Autodesk Fusion 360 part; units mm, degrees
(part 2 of 8)
  spline S13 degree 5 poles (-65.8949, -9.4893) (-65.8986, -9.4803) (-65.9059, -9.4622) (-65.917, -9.4352) (-65.9319, -9.3993) (-65.9507, -9.3546) (-65.9697, -9.3101) (-65.9889, -9.2657) (-66.0083, -9.2215) (-66.028, -9.1775) (-66.0478, -9.1337) (-66.0678, -9.09) (-66.088, -9.0466) (-66.1085, -9.0033) (-66.1291, -8.9602) (-66.1499, -8.9173) (-66.171, -8.8746) (-66.1922, -8.8321) (-66.2136, -8.7898) (-66.2353, -8.7476) (-66.2571, -8.7057) (-66.2792, -8.664) (-66.3015, -8.6224) (-66.3239, -8.5811) (-66.3466, -8.54) (-66.3695, -8.4991) (-66.3926, -8.4584) (-66.4159, -8.418) (-66.4394, -8.3777) (-66.4631, -8.3377) (-66.487, -8.2979) (-66.5111, -8.2583) (-66.5355, -8.2189) (-66.56, -8.1798) (-66.5848, -8.1409) (-66.6097, -8.1023) (-66.6349, -8.0638) (-66.6603, -8.0257) (-66.686, -7.9877) (-66.7118, -7.9501) (-66.7378, -7.9127) (-66.7641, -7.8755) (-66.7906, -7.8386) (-66.8173, -7.802) (-66.8443, -7.7657) (-66.8715, -7.7296) (-66.8989, -7.6938) (-66.9265, -7.6583) (-66.9543, -7.6231) (-66.9824, -7.5882) (-67.0107, -7.5535) (-67.0393, -7.5192) (-67.0681, -7.4853) (-67.0972, -7.4517) (-67.1265, -7.4185) (-67.1561, -7.3855) (-67.1859, -7.3529) (-67.216, -7.3206) (-67.2462, -7.2886) (-67.2768, -7.257) (-67.3076, -7.2258) (-67.3388, -7.1952) (-67.3704, -7.1651) (-67.4024, -7.1356) (-67.4347, -7.1066) (-67.4673, -7.078) (-67.5, -7.0497) (-67.5329, -7.0216) (-67.5661, -6.994) (-67.5997, -6.9671) (-67.6341, -6.9414) (-67.6624, -6.9221) (-67.6843, -6.9086) (-67.6991, -6.8999) (-67.7066, -6.8957) knots -1 -1 -1 -1 -1 -1 -0.98571429 -0.97142857 -0.95714286 -0.94285714 -0.92857143 -0.91428571 -0.9 -0.88571429 -0.87142857 -0.85714286 -0.84285714 -0.82857143 -0.81428571 -0.8 -0.78571429 -0.77142857 -0.75714286 -0.74285714 -0.72857143 -0.71428571 -0.7 -0.68571429 -0.67142857 -0.65714286 -0.64285714 -0.62857143 -0.61428571 -0.6 -0.58571429 -0.57142857 -0.55714286 -0.54285714 -0.52857143 -0.51428571 -0.5 -0.48571429 -0.47142857 -0.45714286 -0.44285714 -0.42857143 -0.41428571 -0.4 -0.38571429 -0.37142857 -0.35714286 -0.34285714 -0.32857143 -0.31428571 -0.3 -0.28571429 -0.27142857 -0.25714286 -0.24285714 -0.22857143 -0.21428571 -0.2 -0.18571429 -0.17142857 -0.15714286 -0.14285714 -0.12857143 -0.11428571 -0.1 -0.08571429 -0.07142857 -0.05714286 -0.04285714 -0.02857143 -0.01428571 0 0 0 0 0 0
  arc A44 (-68.6316, -5.3144) -> (-68.4437, -4.8923) centre (-80, 0) ccw
  spline S14 degree 5 poles (-66.6495, -4.5217) (-66.6414, -4.5244) (-66.6251, -4.5297) (-66.6004, -4.5368) (-66.5672, -4.545) (-66.525, -4.5533) (-66.4826, -4.5603) (-66.4398, -4.5664) (-66.397, -4.5721) (-66.354, -4.5775) (-66.3109, -4.5826) (-66.2678, -4.5872) (-66.2244, -4.5912) (-66.1809, -4.5946) (-66.1373, -4.5973) (-66.0935, -4.5993) (-66.0496, -4.6009) (-66.0055, -4.602) (-65.9614, -4.6027) (-65.9172, -4.603) (-65.873, -4.6029) (-65.8286, -4.6025) (-65.7842, -4.6016) (-65.7397, -4.6003) (-65.6951, -4.5986) (-65.6504, -4.5965) (-65.6057, -4.594) (-65.5609, -4.5911) (-65.516, -4.5879) (-65.4711, -4.5843) (-65.4261, -4.5803) (-65.381, -4.5761) (-65.336, -4.5714) (-65.2908, -4.5664) (-65.2456, -4.5611) (-65.2004, -4.5554) (-65.1551, -4.5494) (-65.1098, -4.5431) (-65.0644, -4.5364) (-65.019, -4.5294) (-64.9736, -4.5221) (-64.9281, -4.5145) (-64.8826, -4.5066) (-64.8371, -4.4983) (-64.7915, -4.4898) (-64.7459, -4.4809) (-64.7003, -4.4717) (-64.6547, -4.4623) (-64.609, -4.4525) (-64.5633, -4.4424) (-64.5176, -4.4321) (-64.4719, -4.4214) (-64.4262, -4.4105) (-64.3804, -4.3992) (-64.3346, -4.3877) (-64.2889, -4.3759) (-64.2431, -4.3638) (-64.1973, -4.3514) (-64.1515, -4.3387) (-64.1056, -4.3258) (-64.0598, -4.3125) (-64.014, -4.299) (-63.9682, -4.2853) (-63.9223, -4.2712) (-63.8765, -4.2569) (-63.8307, -4.2423) (-63.7848, -4.2274) (-63.739, -4.2123) (-63.6932, -4.1969) (-63.6474, -4.1812) (-63.6015, -4.1653) (-63.5649, -4.1523) (-63.5374, -4.1425) (-63.5191, -4.1359) (-63.5099, -4.1325) knots 0 0 0 0 0 0 0.01428571 0.02857143 0.04285714 0.05714286 0.07142857 0.08571429 0.1 0.11428571 0.12857143 0.14285714 0.15714286 0.17142857 0.18571429 0.2 0.21428571 0.22857143 0.24285714 0.25714286 0.27142857 0.28571429 0.3 0.31428571 0.32857143 0.34285714 0.35714286 0.37142857 0.38571429 0.4 0.41428571 0.42857143 0.44285714 0.45714286 0.47142857 0.48571429 0.5 0.51428571 0.52857143 0.54285714 0.55714286 0.57142857 0.58571429 0.6 0.61428571 0.62857143 0.64285714 0.65714286 0.67142857 0.68571429 0.7 0.71428571 0.72857143 0.74285714 0.75714286 0.77142857 0.78571429 0.8 0.81428571 0.82857143 0.84285714 0.85714286 0.87142857 0.88571429 0.9 0.91428571 0.92857143 0.94285714 0.95714286 0.97142857 0.98571429 1 1 1 1 1 1
  arc A45 (-63.5099, -4.1325) -> (-63.2547, -2.9318) centre (-80, 0) ccw
  spline S15 degree 5 poles (-63.2547, -2.9318) (-63.2617, -2.9251) (-63.2758, -2.9116) (-63.2969, -2.8914) (-63.3251, -2.8647) (-63.3605, -2.8315) (-63.3959, -2.7985) (-63.4315, -2.7658) (-63.4673, -2.7334) (-63.5031, -2.7011) (-63.539, -2.6692) (-63.5751, -2.6374) (-63.6112, -2.606) (-63.6475, -2.5747) (-63.6838, -2.5437) (-63.7203, -2.513) (-63.7569, -2.4826) (-63.7936, -2.4524) (-63.8304, -2.4224) (-63.8673, -2.3927) (-63.9043, -2.3633) (-63.9415, -2.3342) (-63.9787, -2.3053) (-64.016, -2.2767) (-64.0535, -2.2484) (-64.091, -2.2203) (-64.1286, -2.1925) (-64.1664, -2.165) (-64.2042, -2.1378) (-64.2422, -2.1109) (-64.2802, -2.0842) (-64.3184, -2.0579) (-64.3566, -2.0318) (-64.3949, -2.0061) (-64.4334, -1.9806) (-64.4719, -1.9555) (-64.5105, -1.9306) (-64.5493, -1.9061) (-64.5881, -1.8819) (-64.627, -1.858) (-64.666, -1.8344) (-64.7052, -1.8111) (-64.7444, -1.7882) (-64.7837, -1.7656) (-64.8231, -1.7434) (-64.8626, -1.7215) (-64.9021, -1.6999) (-64.9418, -1.6787) (-64.9816, -1.6579) (-65.0214, -1.6374) (-65.0614, -1.6173) (-65.1014, -1.5976) (-65.1416, -1.5783) (-65.1818, -1.5594) (-65.2221, -1.541) (-65.2626, -1.5229) (-65.3031, -1.5053) (-65.3436, -1.4879) (-65.3843, -1.471) (-65.4251, -1.4546) (-65.4659, -1.4387) (-65.5069, -1.4234) (-65.548, -1.4088) (-65.5892, -1.3948) (-65.6305, -1.3815) (-65.6719, -1.3686) (-65.7134, -1.356) (-65.7548, -1.3438) (-65.7964, -1.332) (-65.838, -1.3211) (-65.8799, -1.3116) (-65.9136, -1.3055) (-65.939, -1.302) (-65.9561, -1.3002) (-65.9646, -1.2994) knots -1 -1 -1 -1 -1 -1 -0.98571429 -0.97142857 -0.95714286 -0.94285714 -0.92857143 -0.91428571 -0.9 -0.88571429 -0.87142857 -0.85714286 -0.84285714 -0.82857143 -0.81428571 -0.8 -0.78571429 -0.77142857 -0.75714286 -0.74285714 -0.72857143 -0.71428571 -0.7 -0.68571429 -0.67142857 -0.65714286 -0.64285714 -0.62857143 -0.61428571 -0.6 -0.58571429 -0.57142857 -0.55714286 -0.54285714 -0.52857143 -0.51428571 -0.5 -0.48571429 -0.47142857 -0.45714286 -0.44285714 -0.42857143 -0.41428571 -0.4 -0.38571429 -0.37142857 -0.35714286 -0.34285714 -0.32857143 -0.31428571 -0.3 -0.28571429 -0.27142857 -0.25714286 -0.24285714 -0.22857143 -0.21428571 -0.2 -0.18571429 -0.17142857 -0.15714286 -0.14285714 -0.12857143 -0.11428571 -0.1 -0.08571429 -0.07142857 -0.05714286 -0.04285714 -0.02857143 -0.01428571 0 0 0 0 0 0
  arc A46 (-67.4529, -0.231) -> (-67.4529, 0.231) centre (-80, 0) ccw
  spline S16 degree 5 poles (-65.9646, 1.2994) (-65.9561, 1.3002) (-65.939, 1.302) (-65.9136, 1.3055) (-65.8799, 1.3116) (-65.838, 1.3211) (-65.7964, 1.332) (-65.7548, 1.3438) (-65.7134, 1.356) (-65.6719, 1.3686) (-65.6305, 1.3815) (-65.5892, 1.3948) (-65.548, 1.4088) (-65.5069, 1.4234) (-65.4659, 1.4387) (-65.4251, 1.4546) (-65.3843, 1.471) (-65.3436, 1.4879) (-65.3031, 1.5053) (-65.2626, 1.5229) (-65.2221, 1.541) (-65.1818, 1.5594) (-65.1416, 1.5783) (-65.1014, 1.5976) (-65.0614, 1.6173) (-65.0214, 1.6374) (-64.9816, 1.6579) (-64.9418, 1.6787) (-64.9021, 1.6999) (-64.8626, 1.7215) (-64.8231, 1.7434) (-64.7837, 1.7656) (-64.7444, 1.7882) (-64.7052, 1.8111) (-64.666, 1.8344) (-64.627, 1.858) (-64.5881, 1.8819) (-64.5493, 1.9061) (-64.5105, 1.9306) (-64.4719, 1.9555) (-64.4334, 1.9806) (-64.3949, 2.0061) (-64.3566, 2.0318) (-64.3184, 2.0579) (-64.2802, 2.0842) (-64.2422, 2.1109) (-64.2042, 2.1378) (-64.1664, 2.165) (-64.1286, 2.1925) (-64.091, 2.2203) (-64.0535, 2.2484) (-64.016, 2.2767) (-63.9787, 2.3053) (-63.9415, 2.3342) (-63.9043, 2.3633) (-63.8673, 2.3927) (-63.8304, 2.4224) (-63.7936, 2.4524) (-63.7569, 2.4826) (-63.7203, 2.513) (-63.6838, 2.5437) (-63.6475, 2.5747) (-63.6112, 2.606) (-63.5751, 2.6374) (-63.539, 2.6692) (-63.5031, 2.7011) (-63.4673, 2.7334) (-63.4315, 2.7658) (-63.3959, 2.7985) (-63.3605, 2.8315) (-63.3251, 2.8647) (-63.2969, 2.8914) (-63.2758, 2.9116) (-63.2617, 2.9251) (-63.2547, 2.9318) knots 0 0 0 0 0 0 0.01428571 0.02857143 0.04285714 0.05714286 0.07142857 0.08571429 0.1 0.11428571 0.12857143 0.14285714 0.15714286 0.17142857 0.18571429 0.2 0.21428571 0.22857143 0.24285714 0.25714286 0.27142857 0.28571429 0.3 0.31428571 0.32857143 0.34285714 0.35714286 0.37142857 0.38571429 0.4 0.41428571 0.42857143 0.44285714 0.45714286 0.47142857 0.48571429 0.5 0.51428571 0.52857143 0.54285714 0.55714286 0.57142857 0.58571429 0.6 0.61428571 0.62857143 0.64285714 0.65714286 0.67142857 0.68571429 0.7 0.71428571 0.72857143 0.74285714 0.75714286 0.77142857 0.78571429 0.8 0.81428571 0.82857143 0.84285714 0.85714286 0.87142857 0.88571429 0.9 0.91428571 0.92857143 0.94285714 0.95714286 0.97142857 0.98571429 1 1 1 1 1 1
  arc A47 (-63.2547, 2.9318) -> (-63.5099, 4.1325) centre (-80, 0) ccw
  spline S17 degree 5 poles (-63.5099, 4.1325) (-63.5191, 4.1359) (-63.5374, 4.1425) (-63.5649, 4.1523) (-63.6015, 4.1653) (-63.6474, 4.1812) (-63.6932, 4.1969) (-63.739, 4.2123) (-63.7848, 4.2274) (-63.8307, 4.2423) (-63.8765, 4.2569) (-63.9223, 4.2712) (-63.9682, 4.2853) (-64.014, 4.299) (-64.0598, 4.3125) (-64.1056, 4.3258) (-64.1515, 4.3387) (-64.1973, 4.3514) (-64.2431, 4.3638) (-64.2889, 4.3759) (-64.3346, 4.3877) (-64.3804, 4.3992) (-64.4262, 4.4105) (-64.4719, 4.4214) (-64.5176, 4.4321) (-64.5633, 4.4424) (-64.609, 4.4525) (-64.6547, 4.4623) (-64.7003, 4.4717) (-64.7459, 4.4809) (-64.7915, 4.4898) (-64.8371, 4.4983) (-64.8826, 4.5066) (-64.9281, 4.5145) (-64.9736, 4.5221) (-65.019, 4.5294) (-65.0644, 4.5364) (-65.1098, 4.5431) (-65.1551, 4.5494) (-65.2004, 4.5554) (-65.2456, 4.5611) (-65.2908, 4.5664) (-65.336, 4.5714) (-65.381, 4.5761) (-65.4261, 4.5803) (-65.4711, 4.5843) (-65.516, 4.5879) (-65.5609, 4.5911) (-65.6057, 4.594) (-65.6504, 4.5965) (-65.6951, 4.5986) (-65.7397, 4.6003) (-65.7842, 4.6016) (-65.8286, 4.6025) (-65.873, 4.6029) (-65.9172, 4.603) (-65.9614, 4.6027) (-66.0055, 4.602) (-66.0496, 4.6009) (-66.0935, 4.5993) (-66.1373, 4.5973) (-66.1809, 4.5946) (-66.2244, 4.5912) (-66.2678, 4.5872) (-66.3109, 4.5826) (-66.354, 4.5775) (-66.397, 4.5721) (-66.4398, 4.5664) (-66.4826, 4.5603) (-66.525, 4.5533) (-66.5672, 4.545) (-66.6004, 4.5368) (-66.6251, 4.5297) (-66.6414, 4.5244) (-66.6495, 4.5217) knots -1 -1 -1 -1 -1 -1 -0.98571429 -0.97142857 -0.95714286 -0.94285714 -0.92857143 -0.91428571 -0.9 -0.88571429 -0.87142857 -0.85714286 -0.84285714 -0.82857143 -0.81428571 -0.8 -0.78571429 -0.77142857 -0.75714286 -0.74285714 -0.72857143 -0.71428571 -0.7 -0.68571429 -0.67142857 -0.65714286 -0.64285714 -0.62857143 -0.61428571 -0.6 -0.58571429 -0.57142857 -0.55714286 -0.54285714 -0.52857143 -0.51428571 -0.5 -0.48571429 -0.47142857 -0.45714286 -0.44285714 -0.42857143 -0.41428571 -0.4 -0.38571429 -0.37142857 -0.35714286 -0.34285714 -0.32857143 -0.31428571 -0.3 -0.28571429 -0.27142857 -0.25714286 -0.24285714 -0.22857143 -0.21428571 -0.2 -0.18571429 -0.17142857 -0.15714286 -0.14285714 -0.12857143 -0.11428571 -0.1 -0.08571429 -0.07142857 -0.05714286 -0.04285714 -0.02857143 -0.01428571 0 0 0 0 0 0
  arc A48 (-68.4437, 4.8923) -> (-68.6316, 5.3144) centre (-80, 0) ccw
  spline S18 degree 5 poles (-67.7066, 6.8957) (-67.6991, 6.8999) (-67.6843, 6.9086) (-67.6624, 6.9221) (-67.6341, 6.9414) (-67.5997, 6.9671) (-67.5661, 6.994) (-67.5329, 7.0216) (-67.5, 7.0497) (-67.4673, 7.078) (-67.4347, 7.1066) (-67.4024, 7.1356) (-67.3704, 7.1651) (-67.3388, 7.1952) (-67.3076, 7.2258) (-67.2768, 7.257) (-67.2462, 7.2886) (-67.216, 7.3206) (-67.1859, 7.3529) (-67.1561, 7.3855) (-67.1265, 7.4185) (-67.0972, 7.4517) (-67.0681, 7.4853) (-67.0393, 7.5192) (-67.0107, 7.5535) (-66.9824, 7.5882) (-66.9543, 7.6231) (-66.9265, 7.6583) (-66.8989, 7.6938) (-66.8715, 7.7296) (-66.8443, 7.7657) (-66.8173, 7.802) (-66.7906, 7.8386) (-66.7641, 7.8755) (-66.7378, 7.9127) (-66.7118, 7.9501) (-66.686, 7.9877) (-66.6603, 8.0257) (-66.6349, 8.0638) (-66.6097, 8.1023) (-66.5848, 8.1409) (-66.56, 8.1798) (-66.5355, 8.2189) (-66.5111, 8.2583) (-66.487, 8.2979) (-66.4631, 8.3377) (-66.4394, 8.3777) (-66.4159, 8.418) (-66.3926, 8.4584) (-66.3695, 8.4991) (-66.3466, 8.54) (-66.3239, 8.5811) (-66.3015, 8.6224) (-66.2792, 8.664) (-66.2571, 8.7057) (-66.2353, 8.7476) (-66.2136, 8.7898) (-66.1922, 8.8321) (-66.171, 8.8746) (-66.1499, 8.9173) (-66.1291, 8.9602) (-66.1085, 9.0033) (-66.088, 9.0466) (-66.0678, 9.09) (-66.0478, 9.1337) (-66.028, 9.1775) (-66.0083, 9.2215) (-65.9889, 9.2657) (-65.9697, 9.3101) (-65.9507, 9.3546) (-65.9319, 9.3993) (-65.917, 9.4352) (-65.9059, 9.4622) (-65.8986, 9.4803) (-65.8949, 9.4893) knots 0 0 0 0 0 0 0.01428571 0.02857143 0.04285714 0.05714286 0.07142857 0.08571429 0.1 0.11428571 0.12857143 0.14285714 0.15714286 0.17142857 0.18571429 0.2 0.21428571 0.22857143 0.24285714 0.25714286 0.27142857 0.28571429 0.3 0.31428571 0.32857143 0.34285714 0.35714286 0.37142857 0.38571429 0.4 0.41428571 0.42857143 0.44285714 0.45714286 0.47142857 0.48571429 0.5 0.51428571 0.52857143 0.54285714 0.55714286 0.57142857 0.58571429 0.6 0.61428571 0.62857143 0.64285714 0.65714286 0.67142857 0.68571429 0.7 0.71428571 0.72857143 0.74285714 0.75714286 0.77142857 0.78571429 0.8 0.81428571 0.82857143 0.84285714 0.85714286 0.87142857 0.88571429 0.9 0.91428571 0.92857143 0.94285714 0.95714286 0.97142857 0.98571429 1 1 1 1 1 1
  arc A49 (-65.8949, 9.4893) -> (-66.6164, 10.4824) centre (-80, 0) ccw
  spline S19 degree 5 poles (-66.6164, 10.4824) (-66.6262, 10.4817) (-66.6456, 10.4803) (-66.6747, 10.4781) (-66.7134, 10.475) (-66.7618, 10.4709) (-66.81, 10.4666) (-66.8581, 10.4621) (-66.9061, 10.4572) (-66.9541, 10.4522) (-67.0019, 10.4469) (-67.0496, 10.4413) (-67.0972, 10.4355) (-67.1446, 10.4295) (-67.192, 10.4232) (-67.2392, 10.4166) (-67.2864, 10.4098) (-67.3334, 10.4027) (-67.3802, 10.3954) (-67.427, 10.3879) (-67.4736, 10.38) (-67.5201, 10.3719) (-67.5665, 10.3636) (-67.6127, 10.355) (-67.6588, 10.3461) (-67.7048, 10.337) (-67.7506, 10.3276) (-67.7963, 10.318) (-67.8419, 10.3081) (-67.8873, 10.2979) (-67.9325, 10.2875) (-67.9776, 10.2767) (-68.0226, 10.2658) (-68.0674, 10.2545) (-68.112, 10.243) (-68.1565, 10.2312) (-68.2008, 10.2191) (-68.245, 10.2067) (-68.2889, 10.1941) (-68.3327, 10.1811) (-68.3764, 10.1679) (-68.4198, 10.1544) (-68.4631, 10.1406) (-68.5062, 10.1265) (-68.5491, 10.1121) (-68.5918, 10.0974) (-68.6343, 10.0824) (-68.6766, 10.0671) (-68.7187, 10.0515) (-68.7606, 10.0356) (-68.8022, 10.0194) (-68.8437, 10.0028) (-68.8849, 9.9859) (-68.9258, 9.9686) (-68.9665, 9.951) (-69.007, 9.933) (-69.0472, 9.9147) (-69.0872, 9.8962) (-69.127, 9.8773) (-69.1665, 9.858) (-69.2057, 9.8383) (-69.2444, 9.8181) (-69.2828, 9.7973) (-69.3207, 9.776) (-69.3583, 9.7542) (-69.3956, 9.7321) (-69.4327, 9.7097) (-69.4695, 9.6871) (-69.506, 9.6641) (-69.542, 9.6404) (-69.5771, 9.6157) (-69.6042, 9.5947) (-69.6238, 9.5781) (-69.6366, 9.5667) (-69.6429, 9.5609) knots -1 -1 -1 -1 -1 -1 -0.98571429 -0.97142857 -0.95714286 -0.94285714 -0.92857143 -0.91428571 -0.9 -0.88571429 -0.87142857 -0.85714286 -0.84285714 -0.82857143 -0.81428571 -0.8 -0.78571429 -0.77142857 -0.75714286 -0.74285714 -0.72857143 -0.71428571 -0.7 -0.68571429 -0.67142857 -0.65714286 -0.64285714 -0.62857143 -0.61428571 -0.6 -0.58571429 -0.57142857 -0.55714286 -0.54285714 -0.52857143 -0.51428571 -0.5 -0.48571429 -0.47142857 -0.45714286 -0.44285714 -0.42857143 -0.41428571 -0.4 -0.38571429 -0.37142857 -0.35714286 -0.34285714 -0.32857143 -0.31428571 -0.3 -0.28571429 -0.27142857 -0.25714286 -0.24285714 -0.22857143 -0.21428571 -0.2 -0.18571429 -0.17142857 -0.15714286 -0.14285714 -0.12857143 -0.11428571 -0.1 -0.08571429 -0.07142857 -0.05714286 -0.04285714 -0.02857143 -0.01428571 0 0 0 0 0 0
  arc A50 (-71.4327, 9.1697) -> (-71.7761, 9.4789) centre (-80, 0) ccw
  spline S20 degree 5 poles (-71.5741, 11.2998) (-71.569, 11.3066) (-71.559, 11.3205) (-71.5445, 11.3418) (-71.5265, 11.3709) (-71.5055, 11.4084) (-71.4858, 11.4466) (-71.4667, 11.4854) (-71.4481, 11.5244) (-71.4297, 11.5636) (-71.4116, 11.603) (-71.3939, 11.6426) (-71.3766, 11.6826) (-71.36, 11.7229) (-71.3439, 11.7636) (-71.3284, 11.8046) (-71.3134, 11.8459) (-71.2987, 11.8874) (-71.2844, 11.9292) (-71.2705, 11.9711) (-71.2569, 12.0132) (-71.2436, 12.0555) (-71.2307, 12.098) (-71.2181, 12.1408) (-71.206, 12.1837) (-71.1942, 12.2269) (-71.1828, 12.2702) (-71.1717, 12.3137) (-71.1609, 12.3574) (-71.1504, 12.4012) (-71.1402, 12.4452) (-71.1304, 12.4894) (-71.1209, 12.5337) (-71.1117, 12.5782) (-71.1028, 12.6228) (-71.0942, 12.6676) (-71.0859, 12.7125) (-71.0779, 12.7575) (-71.0703, 12.8027) (-71.0629, 12.8481) (-71.0558, 12.8935) (-71.049, 12.9391) (-71.0425, 12.9849) (-71.0362, 13.0307) (-71.0303, 13.0767) (-71.0246, 13.1228) (-71.0193, 13.169) (-71.0142, 13.2154) (-71.0093, 13.2618) (-71.0048, 13.3084) (-71.0005, 13.355) (-70.9965, 13.4018) (-70.9928, 13.4487) (-70.9894, 13.4957) (-70.9862, 13.5428) (-70.9833, 13.59) (-70.9806, 13.6373) (-70.9783, 13.6846) (-70.9762, 13.7321) (-70.9743, 13.7797) (-70.9727, 13.8274) (-70.9714, 13.8751) (-70.9704, 13.923) (-70.9696, 13.9709) (-70.969, 14.0189) (-70.9687, 14.067) (-70.9687, 14.1152) (-70.969, 14.1635) (-70.9694, 14.2118) (-70.9702, 14.2602) (-70.9712, 14.3087) (-70.9722, 14.3476) (-70.9731, 14.3768) (-70.9737, 14.3962) (-70.974, 14.406) knots 0 0 0 0 0 0 0.01428571 0.02857143 0.04285714 0.05714286 0.07142857 0.08571429 0.1 0.11428571 0.12857143 0.14285714 0.15714286 0.17142857 0.18571429 0.2 0.21428571 0.22857143 0.24285714 0.25714286 0.27142857 0.28571429 0.3 0.31428571 0.32857143 0.34285714 0.35714286 0.37142857 0.38571429 0.4 0.41428571 0.42857143 0.44285714 0.45714286 0.47142857 0.48571429 0.5 0.51428571 0.52857143 0.54285714 0.55714286 0.57142857 0.58571429 0.6 0.61428571 0.62857143 0.64285714 0.65714286 0.67142857 0.68571429 0.7 0.71428571 0.72857143 0.74285714 0.75714286 0.77142857 0.78571429 0.8 0.81428571 0.82857143 0.84285714 0.85714286 0.87142857 0.88571429 0.9 0.91428571 0.92857143 0.94285714 0.95714286 0.97142857 0.98571429 1 1 1 1 1 1
  arc A51 (-70.974, 14.406) -> (-72.0371, 15.0197) centre (-80, 0) ccw
  spline S21 degree 5 poles (-72.0371, 15.0197) (-72.0457, 15.0151) (-72.0628, 15.0059) (-72.0885, 14.9921) (-72.1227, 14.9735) (-72.1652, 14.9502) (-72.2075, 14.9266) (-72.2496, 14.9028) (-72.2915, 14.8789) (-72.3332, 14.8548) (-72.3748, 14.8305) (-72.4161, 14.806) (-72.4572, 14.7814) (-72.4981, 14.7565) (-72.5388, 14.7315) (-72.5793, 14.7063) (-72.6196, 14.6809) (-72.6596, 14.6554) (-72.6995, 14.6296) (-72.7391, 14.6037) (-72.7785, 14.5776) (-72.8177, 14.5513) (-72.8567, 14.5248) (-72.8954, 14.4981) (-72.9339, 14.4713) (-72.9722, 14.4443) (-73.0103, 14.417) (-73.0481, 14.3896) (-73.0857, 14.3621) (-73.123, 14.3343) (-73.1601, 14.3063) (-73.1969, 14.2782) (-73.2335, 14.2499) (-73.2699, 14.2214) (-73.306, 14.1927) (-73.3418, 14.1638) (-73.3774, 14.1348) (-73.4127, 14.1055) (-73.4477, 14.0761) (-73.4825, 14.0464) (-73.517, 14.0166) (-73.5512, 13.9866) (-73.5851, 13.9564) (-73.6187, 13.926) (-73.652, 13.8954) (-73.685, 13.8646) (-73.7178, 13.8336) (-73.7502, 13.8024) (-73.7823, 13.7711) (-73.8141, 13.7395) (-73.8456, 13.7077) (-73.8767, 13.6757) (-73.9075, 13.6435) (-73.9378, 13.611) (-73.9678, 13.5784) (-73.9975, 13.5455) (-74.0268, 13.5125) (-74.0558, 13.4792) (-74.0845, 13.4458) (-74.1127, 13.4121) (-74.1405, 13.3782) (-74.1677, 13.3439) (-74.1943, 13.3094) (-74.2203, 13.2745) (-74.2457, 13.2393) (-74.2708, 13.2039) (-74.2956, 13.1684) (-74.32, 13.1327) (-74.344, 13.0969) (-74.3673, 13.0606) (-74.3893, 13.0237) (-74.4054, 12.9935) (-74.4166, 12.9704) (-74.4237, 12.9548) (-74.4271, 12.9469) knots -1 -1 -1 -1 -1 -1 -0.98571429 -0.97142857 -0.95714286 -0.94285714 -0.92857143 -0.91428571 -0.9 -0.88571429 -0.87142857 -0.85714286 -0.84285714 -0.82857143 -0.81428571 -0.8 -0.78571429 -0.77142857 -0.75714286 -0.74285714 -0.72857143 -0.71428571 -0.7 -0.68571429 -0.67142857 -0.65714286 -0.64285714 -0.62857143 -0.61428571 -0.6 -0.58571429 -0.57142857 -0.55714286 -0.54285714 -0.52857143 -0.51428571 -0.5 -0.48571429 -0.47142857 -0.45714286 -0.44285714 -0.42857143 -0.41428571 -0.4 -0.38571429 -0.37142857 -0.35714286 -0.34285714 -0.32857143 -0.31428571 -0.3 -0.28571429 -0.27142857 -0.25714286 -0.24285714 -0.22857143 -0.21428571 -0.2 -0.18571429 -0.17142857 -0.15714286 -0.14285714 -0.12857143 -0.11428571 -0.1 -0.08571429 -0.07142857 -0.05714286 -0.04285714 -0.02857143 -0.01428571 0 0 0 0 0 0
  arc A52 (-75.903, 11.8616) -> (-76.3425, 12.0044) centre (-80, 0) ccw
  spline S22 degree 5 poles (-76.8986, 13.75) (-76.8967, 13.7583) (-76.8932, 13.7751) (-76.8887, 13.8004) (-76.884, 13.8343) (-76.8801, 13.8771) (-76.8776, 13.9201) (-76.876, 13.9632) (-76.8748, 14.0064) (-76.874, 14.0497) (-76.8734, 14.0931) (-76.8734, 14.1365) (-76.8739, 14.18) (-76.8751, 14.2236) (-76.877, 14.2673) (-76.8795, 14.3111) (-76.8825, 14.3549) (-76.8861, 14.3988) (-76.89, 14.4428) (-76.8943, 14.4867) (-76.8989, 14.5308) (-76.904, 14.5748) (-76.9095, 14.6189) (-76.9155, 14.6631) (-76.9218, 14.7072) (-76.9286, 14.7514) (-76.9358, 14.7957) (-76.9433, 14.8399) (-76.9512, 14.8842) (-76.9595, 14.9285) (-76.9681, 14.9729) (-76.9771, 15.0172) (-76.9864, 15.0616) (-76.9961, 15.1059) (-77.0061, 15.1503) (-77.0165, 15.1947) (-77.0272, 15.2391) (-77.0383, 15.2835) (-77.0496, 15.3279) (-77.0613, 15.3724) (-77.0733, 15.4168) (-77.0857, 15.4612) (-77.0983, 15.5056) (-77.1113, 15.5501) (-77.1245, 15.5945) (-77.1381, 15.6389) (-77.152, 15.6833) (-77.1662, 15.7277) (-77.1807, 15.7721) (-77.1955, 15.8165) (-77.2106, 15.8608) (-77.2259, 15.9052) (-77.2416, 15.9495) (-77.2576, 15.9939) (-77.2738, 16.0382) (-77.2904, 16.0825) (-77.3072, 16.1268) (-77.3243, 16.171) (-77.3417, 16.2152) (-77.3593, 16.2595) (-77.3773, 16.3036) (-77.3955, 16.3478) (-77.414, 16.3919) (-77.4328, 16.4361) (-77.4518, 16.4801) (-77.4711, 16.5242) (-77.4907, 16.5682) (-77.5105, 16.6122) (-77.5306, 16.6562) (-77.551, 16.7001) (-77.5716, 16.744) (-77.5884, 16.7791) (-77.601, 16.8054) (-77.6095, 16.8229) (-77.6138, 16.8317) knots 0 0 0 0 0 0 0.01428571 0.02857143 0.04285714 0.05714286 0.07142857 0.08571429 0.1 0.11428571 0.12857143 0.14285714 0.15714286 0.17142857 0.18571429 0.2 0.21428571 0.22857143 0.24285714 0.25714286 0.27142857 0.28571429 0.3 0.31428571 0.32857143 0.34285714 0.35714286 0.37142857 0.38571429 0.4 0.41428571 0.42857143 0.44285714 0.45714286 0.47142857 0.48571429 0.5 0.51428571 0.52857143 0.54285714 0.55714286 0.57142857 0.58571429 0.6 0.61428571 0.62857143 0.64285714 0.65714286 0.67142857 0.68571429 0.7 0.71428571 0.72857143 0.74285714 0.75714286 0.77142857 0.78571429 0.8 0.81428571 0.82857143 0.84285714 0.85714286 0.87142857 0.88571429 0.9 0.91428571 0.92857143 0.94285714 0.95714286 0.97142857 0.98571429 1 1 1 1 1 1
  arc A53 (-77.6138, 16.8317) -> (-78.8346, 16.96) centre (-80, 0) ccw
  spline S23 degree 5 poles (-78.8346, 16.96) (-78.8406, 16.9523) (-78.8525, 16.9369) (-78.8704, 16.9138) (-78.894, 16.883) (-78.9233, 16.8444) (-78.9524, 16.8056) (-78.9812, 16.7668) (-79.0098, 16.7279) (-79.0381, 16.6889) (-79.0661, 16.6498) (-79.0939, 16.6107) (-79.1214, 16.5714) (-79.1487, 16.5321) (-79.1757, 16.4927) (-79.2024, 16.4532) (-79.2289, 16.4136) (-79.2551, 16.3739) (-79.281, 16.3342) (-79.3067, 16.2944) (-79.3321, 16.2545) (-79.3572, 16.2145) (-79.382, 16.1745) (-79.4066, 16.1344) (-79.4308, 16.0942) (-79.4548, 16.0539) (-79.4785, 16.0136) (-79.5019, 15.9732) (-79.525, 15.9327) (-79.5478, 15.8922) (-79.5704, 15.8515) (-79.5926, 15.8109) (-79.6145, 15.7701) (-79.6361, 15.7293) (-79.6574, 15.6884) (-79.6784, 15.6474) (-79.699, 15.6064) (-79.7194, 15.5653) (-79.7394, 15.5242) (-79.7591, 15.483) (-79.7785, 15.4417) (-79.7975, 15.4004) (-79.8162, 15.359) (-79.8346, 15.3175) (-79.8526, 15.276) (-79.8702, 15.2345) (-79.8875, 15.1928) (-79.9045, 15.1512) (-79.9211, 15.1094) (-79.9373, 15.0677) (-79.9531, 15.0258) (-79.9685, 14.9839) (-79.9835, 14.942) (-79.998, 14.9) (-80.0122, 14.858) (-80.0259, 14.8159) (-80.0392, 14.7738) (-80.0522, 14.7316) (-80.0648, 14.6894) (-80.0769, 14.6471) (-80.0884, 14.6049) (-80.0994, 14.5625) (-80.1096, 14.5201) (-80.1192, 14.4777) (-80.1281, 14.4352) (-80.1366, 14.3927) (-80.1448, 14.3501) (-80.1526, 14.3076) (-80.16, 14.2651) (-80.1665, 14.2225) (-80.1716, 14.1799) (-80.1741, 14.1457) (-80.1749, 14.12) (-80.1749, 14.1029) (-80.1748, 14.0943) knots -1 -1 -1 -1 -1 -1 -0.98571429 -0.97142857 -0.95714286 -0.94285714 -0.92857143 -0.91428571 -0.9 -0.88571429 -0.87142857 -0.85714286 -0.84285714 -0.82857143 -0.81428571 -0.8 -0.78571429 -0.77142857 -0.75714286 -0.74285714 -0.72857143 -0.71428571 -0.7 -0.68571429 -0.67142857 -0.65714286 -0.64285714 -0.62857143 -0.61428571 -0.6 -0.58571429 -0.57142857 -0.55714286 -0.54285714 -0.52857143 -0.51428571 -0.5 -0.48571429 -0.47142857 -0.45714286 -0.44285714 -0.42857143 -0.41428571 -0.4 -0.38571429 -0.37142857 -0.35714286 -0.34285714 -0.32857143 -0.31428571 -0.3 -0.28571429 -0.27142857 -0.25714286 -0.24285714 -0.22857143 -0.21428571 -0.2 -0.18571429 -0.17142857 -0.15714286 -0.14285714 -0.12857143 -0.11428571 -0.1 -0.08571429 -0.07142857 -0.05714286 -0.04285714 -0.02857143 -0.01428571 0 0 0 0 0 0
  arc A54 (-81.0818, 12.5025) -> (-81.5413, 12.4542) centre (-80, 0) ccw
  spline S24 degree 5 poles (-82.7594, 13.8227) (-82.761, 13.8311) (-82.7646, 13.8478) (-82.7708, 13.8728) (-82.7804, 13.9057) (-82.7942, 13.9463) (-82.8094, 13.9866) (-82.8254, 14.0267) (-82.8419, 14.0666) (-82.8588, 14.1065) (-82.8759, 14.1464) (-82.8935, 14.1861) (-82.9117, 14.2256) (-82.9305, 14.2649) (-82.95, 14.3041) (-82.9701, 14.3431) (-82.9907, 14.3819) (-83.0118, 14.4205) (-83.0333, 14.4591) (-83.0551, 14.4975) (-83.0772, 14.5358) (-83.0998, 14.574) (-83.1228, 14.6121) (-83.1461, 14.65) (-83.1699, 14.6877) (-83.1941, 14.7254) (-83.2186, 14.7629) (-83.2435, 14.8002) (-83.2688, 14.8375) (-83.2944, 14.8746) (-83.3203, 14.9116) (-83.3465, 14.9484) (-83.3731, 14.9851) (-83.3999, 15.0217) (-83.4272, 15.0582) (-83.4547, 15.0945) (-83.4825, 15.1308) (-83.5107, 15.1668) (-83.5391, 15.2028) (-83.5679, 15.2386) (-83.5969, 15.2743) (-83.6263, 15.3099) (-83.6559, 15.3453) (-83.6858, 15.3806) (-83.716, 15.4158) (-83.7464, 15.4509) (-83.7772, 15.4858) (-83.8082, 15.5206) (-83.8395, 15.5552) (-83.8711, 15.5898) (-83.9029, 15.6242) (-83.935, 15.6584) (-83.9673, 15.6926) (-84, 15.7266) (-84.0328, 15.7604) (-84.066, 15.7942) (-84.0993, 15.8278) (-84.133, 15.8613) (-84.1668, 15.8946) (-84.201, 15.9278) (-84.2353, 15.9609) (-84.2699, 15.9938) (-84.3048, 16.0266) (-84.3399, 16.0593) (-84.3752, 16.0918) (-84.4107, 16.1242) (-84.4465, 16.1565) (-84.4826, 16.1886) (-84.5188, 16.2206) (-84.5553, 16.2524) (-84.592, 16.2841) (-84.6215, 16.3094) (-84.6438, 16.3283) (-84.6587, 16.3408) (-84.6661, 16.3471) knots 0 0 0 0 0 0 0.01428571 0.02857143 0.04285714 0.05714286 0.07142857 0.08571429 0.1 0.11428571 0.12857143 0.14285714 0.15714286 0.17142857 0.18571429 0.2 0.21428571 0.22857143 0.24285714 0.25714286 0.27142857 0.28571429 0.3 0.31428571 0.32857143 0.34285714 0.35714286 0.37142857 0.38571429 0.4 0.41428571 0.42857143 0.44285714 0.45714286 0.47142857 0.48571429 0.5 0.51428571 0.52857143 0.54285714 0.55714286 0.57142857 0.58571429 0.6 0.61428571 0.62857143 0.64285714 0.65714286 0.67142857 0.68571429 0.7 0.71428571 0.72857143 0.74285714 0.75714286 0.77142857 0.78571429 0.8 0.81428571 0.82857143 0.84285714 0.85714286 0.87142857 0.88571429 0.9 0.91428571 0.92857143 0.94285714 0.95714286 0.97142857 0.98571429 1 1 1 1 1 1
  arc A55 (-84.6661, 16.3471) -> (-85.8336, 15.9678) centre (-80, 0) ccw
  spline S25 degree 5 poles (-85.8336, 15.9678) (-85.8359, 15.9583) (-85.8406, 15.9394) (-85.8475, 15.911) (-85.8566, 15.8732) (-85.8676, 15.826) (-85.8784, 15.7788) (-85.8889, 15.7316) (-85.8992, 15.6845) (-85.9092, 15.6373) (-85.9189, 15.5902) (-85.9284, 15.5431) (-85.9376, 15.4961) (-85.9465, 15.4491) (-85.9551, 15.4021) (-85.9635, 15.3551) (-85.9716, 15.3082) (-85.9794, 15.2613) (-85.9869, 15.2145) (-85.9942, 15.1677) (-86.0011, 15.1209) (-86.0078, 15.0742) (-86.0142, 15.0275) (-86.0203, 14.9809) (-86.0261, 14.9343) (-86.0317, 14.8877) (-86.0369, 14.8413) (-86.0419, 14.7948) (-86.0465, 14.7484) (-86.0509, 14.7021) (-86.0549, 14.6559) (-86.0586, 14.6096) (-86.0621, 14.5635) (-86.0652, 14.5174) (-86.068, 14.4714) (-86.0706, 14.4255) (-86.0728, 14.3796) (-86.0746, 14.3338) (-86.0762, 14.288) (-86.0775, 14.2424) (-86.0784, 14.1968) (-86.0789, 14.1513) (-86.0792, 14.1059) (-86.0791, 14.0605) (-86.0786, 14.0153) (-86.0779, 13.9702) (-86.0767, 13.9251) (-86.0753, 13.8801) (-86.0734, 13.8353) (-86.0713, 13.7905) (-86.0687, 13.7459) (-86.0657, 13.7013) (-86.0624, 13.6569) (-86.0586, 13.6126) (-86.0544, 13.5685) (-86.0498, 13.5245) (-86.0449, 13.4805) (-86.0396, 13.4368) (-86.0339, 13.3931) (-86.0278, 13.3496) (-86.0211, 13.3062) (-86.0139, 13.2631) (-86.006, 13.2202) (-85.9974, 13.1775) (-85.9883, 13.1351) (-85.9788, 13.0928) (-85.969, 13.0506) (-85.9589, 13.0086) (-85.9483, 12.9667) (-85.9369, 12.9252) (-85.9242, 12.8842) (-85.9126, 12.8519) (-85.9029, 12.8282) (-85.896, 12.8125) (-85.8924, 12.8047) knots -1 -1 -1 -1 -1 -1 -0.98571429 -0.97142857 -0.95714286 -0.94285714 -0.92857143 -0.91428571 -0.9 -0.88571429 -0.87142857 -0.85714286 -0.84285714 -0.82857143 -0.81428571 -0.8 -0.78571429 -0.77142857 -0.75714286 -0.74285714 -0.72857143 -0.71428571 -0.7 -0.68571429 -0.67142857 -0.65714286 -0.64285714 -0.62857143 -0.61428571 -0.6 -0.58571429 -0.57142857 -0.55714286 -0.54285714 -0.52857143 -0.51428571 -0.5 -0.48571429 -0.47142857 -0.45714286 -0.44285714 -0.42857143 -0.41428571 -0.4 -0.38571429 -0.37142857 -0.35714286 -0.34285714 -0.32857143 -0.31428571 -0.3 -0.28571429 -0.27142857 -0.25714286 -0.24285714 -0.22857143 -0.21428571 -0.2 -0.18571429 -0.17142857 -0.15714286 -0.14285714 -0.12857143 -0.11428571 -0.1 -0.08571429 -0.07142857 -0.05714286 -0.04285714 -0.02857143 -0.01428571 0 0 0 0 0 0
  arc A56 (-86.0735, 10.9816) -> (-86.4736, 10.7506) centre (-80, 0) ccw
  spline S26 degree 5 poles (-88.143, 11.5053) (-88.1479, 11.5123) (-88.1581, 11.5261) (-88.1738, 11.5464) (-88.1959, 11.5726) (-88.2251, 11.6041) (-88.2554, 11.6347) (-88.2863, 11.6648) (-88.3177, 11.6946) (-88.3493, 11.7242) (-88.3811, 11.7536) (-88.4134, 11.7827) (-88.446, 11.8114) (-88.4792, 11.8397) (-88.513, 11.8676) (-88.5472, 11.895) (-88.5818, 11.922) (-88.6168, 11.9488) (-88.6521, 11.9753) (-88.6876, 12.0015) (-88.7235, 12.0275) (-88.7596, 12.0532) (-88.796, 12.0786) (-88.8328, 12.1038) (-88.8699, 12.1286) (-88.9073, 12.1531) (-88.945, 12.1774) (-88.9829, 12.2014) (-89.0211, 12.2252) (-89.0596, 12.2487) (-89.0983, 12.2719) (-89.1372, 12.2949) (-89.1764, 12.3177) (-89.2159, 12.3402) (-89.2556, 12.3624) (-89.2955, 12.3844) (-89.3357, 12.4062) (-89.3761, 12.4277) (-89.4167, 12.4489) (-89.4575, 12.47) (-89.4986, 12.4908) (-89.5398, 12.5113) (-89.5813, 12.5317) (-89.623, 12.5518) (-89.6649, 12.5716) (-89.707, 12.5913) (-89.7493, 12.6106) (-89.7918, 12.6298) (-89.8345, 12.6487) (-89.8773, 12.6675) (-89.9204, 12.6859) (-89.9637, 12.7042) (-90.0071, 12.7222) (-90.0507, 12.74) (-90.0945, 12.7576) (-90.1385, 12.7749) (-90.1827, 12.7921) (-90.227, 12.809) (-90.2715, 12.8256) (-90.3162, 12.8421) (-90.361, 12.8583) (-90.406, 12.8743) (-90.4512, 12.8901) (-90.4966, 12.9057) (-90.5421, 12.9211) (-90.5877, 12.9362) (-90.6335, 12.9511) (-90.6795, 12.9658) (-90.7256, 12.9803) (-90.7719, 12.9945) (-90.8183, 13.0085) (-90.8556, 13.0196) (-90.8836, 13.0278) (-90.9023, 13.0332) (-90.9117, 13.0359) knots 0 0 0 0 0 0 0.01428571 0.02857143 0.04285714 0.05714286 0.07142857 0.08571429 0.1 0.11428571 0.12857143 0.14285714 0.15714286 0.17142857 0.18571429 0.2 0.21428571 0.22857143 0.24285714 0.25714286 0.27142857 0.28571429 0.3 0.31428571 0.32857143 0.34285714 0.35714286 0.37142857 0.38571429 0.4 0.41428571 0.42857143 0.44285714 0.45714286 0.47142857 0.48571429 0.5 0.51428571 0.52857143 0.54285714 0.55714286 0.57142857 0.58571429 0.6 0.61428571 0.62857143 0.64285714 0.65714286 0.67142857 0.68571429 0.7 0.71428571 0.72857143 0.74285714 0.75714286 0.77142857 0.78571429 0.8 0.81428571 0.82857143 0.84285714 0.85714286 0.87142857 0.88571429 0.9 0.91428571 0.92857143 0.94285714 0.95714286 0.97142857 0.98571429 1 1 1 1 1 1
  arc A57 (-90.9117, 13.0359) -> (-91.8239, 12.2145) centre (-80, 0) ccw
  spline S27 degree 5 poles (-91.8239, 12.2145) (-91.8222, 12.2049) (-91.8188, 12.1858) (-91.8136, 12.1571) (-91.8065, 12.1188) (-91.7974, 12.0712) (-91.788, 12.0237) (-91.7784, 11.9763) (-91.7686, 11.929) (-91.7586, 11.8819) (-91.7483, 11.8349) (-91.7378, 11.7881) (-91.7271, 11.7413) (-91.7161, 11.6948) (-91.7049, 11.6483) (-91.6934, 11.602) (-91.6817, 11.5559) (-91.6698, 11.5099) (-91.6576, 11.464) (-91.6452, 11.4183) (-91.6325, 11.3728) (-91.6196, 11.3274) (-91.6065, 11.2821) (-91.5931, 11.237) (-91.5795, 11.1921) (-91.5656, 11.1473) (-91.5515, 11.1027) (-91.5371, 11.0583) (-91.5225, 11.014) (-91.5076, 10.97) (-91.4925, 10.926) (-91.4771, 10.8823) (-91.4615, 10.8387) (-91.4456, 10.7954) (-91.4295, 10.7522) (-91.4131, 10.7092) (-91.3964, 10.6664) (-91.3795, 10.6238) (-91.3624, 10.5813) (-91.3449, 10.5391) (-91.3272, 10.4971) (-91.3092, 10.4553) (-91.291, 10.4137) (-91.2725, 10.3724) (-91.2537, 10.3312) (-91.2346, 10.2903) (-91.2152, 10.2496) (-91.1956, 10.2091) (-91.1757, 10.1689) (-91.1555, 10.1289) (-91.135, 10.0891) (-91.1142, 10.0496) (-91.093, 10.0104) (-91.0716, 9.9715) (-91.0498, 9.9329) (-91.0277, 9.8945) (-91.0053, 9.8564) (-90.9827, 9.8186) (-90.9597, 9.781) (-90.9364, 9.7437) (-90.9127, 9.7068) (-90.8885, 9.6704) (-90.8639, 9.6344) (-90.8387, 9.5989) (-90.8131, 9.5638) (-90.7872, 9.529) (-90.7611, 9.4945) (-90.7347, 9.4602) (-90.7081, 9.4263) (-90.6808, 9.393) (-90.6525, 9.3607) (-90.6288, 9.336) (-90.6102, 9.3182) (-90.5975, 9.3067) (-90.5911, 9.301) knots -1 -1 -1 -1 -1 -1 -0.98571429 -0.97142857 -0.95714286 -0.94285714 -0.92857143 -0.91428571 -0.9 -0.88571429 -0.87142857 -0.85714286 -0.84285714 -0.82857143 -0.81428571 -0.8 -0.78571429 -0.77142857 -0.75714286 -0.74285714 -0.72857143 -0.71428571 -0.7 -0.68571429 -0.67142857 -0.65714286 -0.64285714 -0.62857143 -0.61428571 -0.6 -0.58571429 -0.57142857 -0.55714286 -0.54285714 -0.52857143 -0.51428571 -0.5 -0.48571429 -0.47142857 -0.45714286 -0.44285714 -0.42857143 -0.41428571 -0.4 -0.38571429 -0.37142857 -0.35714286 -0.34285714 -0.32857143 -0.31428571 -0.3 -0.28571429 -0.27142857 -0.25714286 -0.24285714 -0.22857143 -0.21428571 -0.2 -0.18571429 -0.17142857 -0.15714286 -0.14285714 -0.12857143 -0.11428571 -0.1 -0.08571429 -0.07142857 -0.05714286 -0.04285714 -0.02857143 -0.01428571 0 0 0 0 0 0
  arc A58 (-90.015, 7.5619) -> (-90.2866, 7.1881) centre (-80, 0) ccw
  spline S28 degree 5 poles (-92.1186, 7.1986) (-92.126, 7.2029) (-92.1409, 7.2115) (-92.1635, 7.2236) (-92.1943, 7.2385) (-92.2338, 7.2554) (-92.2739, 7.2711) (-92.3144, 7.286) (-92.3552, 7.3005) (-92.3961, 7.3146) (-92.4372, 7.3285) (-92.4784, 7.342) (-92.52, 7.355) (-92.5618, 7.3673) (-92.604, 7.379) (-92.6464, 7.3902) (-92.689, 7.4008) (-92.7318, 7.411) (-92.7748, 7.4209) (-92.818, 7.4304) (-92.8613, 7.4395) (-92.9048, 7.4483) (-92.9484, 7.4567) (-92.9922, 7.4647) (-93.0362, 7.4723) (-93.0803, 7.4795) (-93.1246, 7.4864) (-93.1691, 7.4929) (-93.2136, 7.499) (-93.2583, 7.5048) (-93.3031, 7.5103) (-93.3481, 7.5155) (-93.3931, 7.5204) (-93.4383, 7.5249) (-93.4836, 7.529) (-93.5291, 7.5329) (-93.5746, 7.5364) (-93.6203, 7.5397) (-93.666, 7.5426) (-93.7119, 7.5452) (-93.7578, 7.5475) (-93.8039, 7.5495) (-93.8501, 7.5512) (-93.8963, 7.5526) (-93.9427, 7.5537) (-93.9891, 7.5545) (-94.0356, 7.555) (-94.0822, 7.5552) (-94.1289, 7.5552) (-94.1757, 7.5548) (-94.2226, 7.5542) (-94.2695, 7.5533) (-94.3165, 7.5521) (-94.3636, 7.5506) (-94.4108, 7.5488) (-94.458, 7.5468) (-94.5053, 7.5445) (-94.5527, 7.5419) (-94.6001, 7.539) (-94.6477, 7.5359) (-94.6952, 7.5325) (-94.7429, 7.5288) (-94.7906, 7.5248) (-94.8383, 7.5206) (-94.8861, 7.5161) (-94.934, 7.5114) (-94.9819, 7.5064) (-95.0299, 7.5011) (-95.0779, 7.4955) (-95.126, 7.4897) (-95.1741, 7.4837) (-95.2126, 7.4786) (-95.2416, 7.4747) (-95.2609, 7.4721) (-95.2705, 7.4707) knots 0 0 0 0 0 0 0.01428571 0.02857143 0.04285714 0.05714286 0.07142857 0.08571429 0.1 0.11428571 0.12857143 0.14285714 0.15714286 0.17142857 0.18571429 0.2 0.21428571 0.22857143 0.24285714 0.25714286 0.27142857 0.28571429 0.3 0.31428571 0.32857143 0.34285714 0.35714286 0.37142857 0.38571429 0.4 0.41428571 0.42857143 0.44285714 0.45714286 0.47142857 0.48571429 0.5 0.51428571 0.52857143 0.54285714 0.55714286 0.57142857 0.58571429 0.6 0.61428571 0.62857143 0.64285714 0.65714286 0.67142857 0.68571429 0.7 0.71428571 0.72857143 0.74285714 0.75714286 0.77142857 0.78571429 0.8 0.81428571 0.82857143 0.84285714 0.85714286 0.87142857 0.88571429 0.9 0.91428571 0.92857143 0.94285714 0.95714286 0.97142857 0.98571429 1 1 1 1 1 1
  arc A59 (-95.2705, 7.4707) -> (-95.7698, 6.3493) centre (-80, 0) ccw
  spline S29 degree 5 poles (-95.7698, 6.3493) (-95.7643, 6.3412) (-95.7534, 6.3251) (-95.7369, 6.301) (-95.7149, 6.269) (-95.6872, 6.2292) (-95.6594, 6.1896) (-95.6313, 6.1502) (-95.6032, 6.111) (-95.5748, 6.072) (-95.5463, 6.0333) (-95.5177, 5.9947) (-95.4888, 5.9564) (-95.4599, 5.9183) (-95.4307, 5.8805) (-95.4014, 5.8428) (-95.372, 5.8054) (-95.3424, 5.7683) (-95.3126, 5.7313) (-95.2827, 5.6946) (-95.2526, 5.6582) (-95.2223, 5.6219) (-95.1919, 5.5859) (-95.1613, 5.5502) (-95.1306, 5.5147) (-95.0997, 5.4794) (-95.0687, 5.4444) (-95.0375, 5.4097) (-95.0061, 5.3752) (-94.9746, 5.341) (-94.9429, 5.307) (-94.9111, 5.2733) (-94.8791, 5.2399) (-94.847, 5.2067) (-94.8147, 5.1738) (-94.7822, 5.1412) (-94.7496, 5.1089) (-94.7168, 5.0768) (-94.6838, 5.0451) (-94.6507, 5.0136) (-94.6175, 4.9824) (-94.5841, 4.9515) (-94.5505, 4.9209) (-94.5167, 4.8907) (-94.4828, 4.8608) (-94.4487, 4.8311) (-94.4145, 4.8018) (-94.3801, 4.7728) (-94.3455, 4.7442) (-94.3108, 4.7158) (-94.2759, 4.6878) (-94.2408, 4.6602) (-94.2056, 4.633) (-94.1702, 4.6062) (-94.1345, 4.5798) (-94.0988, 4.5537) (-94.0628, 4.528) (-94.0267, 4.5027) (-93.9905, 4.4777) (-93.954, 4.4531) (-93.9174, 4.429) (-93.8805, 4.4056) (-93.8433, 4.3827) (-93.8059, 4.3605) (-93.7682, 4.3389) (-93.7304, 4.3176) (-93.6925, 4.2967) (-93.6545, 4.2761) (-93.6163, 4.256) (-93.5778, 4.2367) (-93.5389, 4.2187) (-93.5072, 4.2057) (-93.483, 4.197) (-93.4667, 4.1917) (-93.4585, 4.1891) knots -1 -1 -1 -1 -1 -1 -0.98571429 -0.97142857 -0.95714286 -0.94285714 -0.92857143 -0.91428571 -0.9 -0.88571429 -0.87142857 -0.85714286 -0.84285714 -0.82857143 -0.81428571 -0.8 -0.78571429 -0.77142857 -0.75714286 -0.74285714 -0.72857143 -0.71428571 -0.7 -0.68571429 -0.67142857 -0.65714286 -0.64285714 -0.62857143 -0.61428571 -0.6 -0.58571429 -0.57142857 -0.55714286 -0.54285714 -0.52857143 -0.51428571 -0.5 -0.48571429 -0.47142857 -0.45714286 -0.44285714 -0.42857143 -0.41428571 -0.4 -0.38571429 -0.37142857 -0.35714286 -0.34285714 -0.32857143 -0.31428571 -0.3 -0.28571429 -0.27142857 -0.25714286 -0.24285714 -0.22857143 -0.21428571 -0.2 -0.18571429 -0.17142857 -0.15714286 -0.14285714 -0.12857143 -0.11428571 -0.1 -0.08571429 -0.07142857 -0.05714286 -0.04285714 -0.02857143 -0.01428571 0 0 0 0 0 0
  point P0 (-80, 0)
  dimension "d17" = 3.3
  dimension "d18" = 5.3
  constraint horizontal L30
  constraint vertical L31
  constraint horizontal L32
  constraint vertical L33
  constraint midpoint L35 P0
  constraint coincident P0 A0.centre
  measures "d17" distance of L30.end L31.end
  measures "d18" distance of L30.start L30.end
extrude "Extrude3" cut sketch "Sketch1 (3)" against normal up to surface (5 mm away) contours L30 L31 L32 L33 sketch seen with x (1, 0, 0) y (0, 1, 0) z (0, 0, 1) at (-80, 0, 0) bodies 1 in component "Spur Gear (15 teeth)"